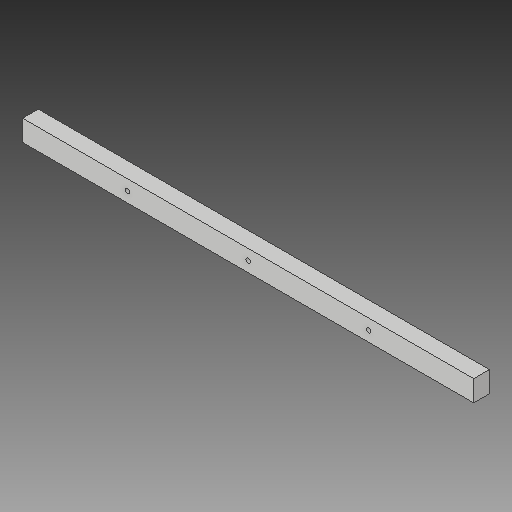
# Autodesk Inventor part: Wiper Springloaded 1
Saved by Autodesk Inventor 2019 (Build 230136000, 136)
## iProperties
Created: 2020-03-14
Part Number: Wiper Springloaded 1
Material: Generic
Document SubType Name: Modeling
Designer: Vijay
Density: 1 g/cm^3
Appearance: Default
Author: Vijay
Autodesk Inventor part; units mm, degrees
ref_plane "YZ Plane" through (0, 0, 0) normal (1, 0, 0) x (0, 1, 0)
ref_plane "XZ Plane" through (0, 0, 0) normal (0, 1, 0) x (-1, 0, 0)
ref_plane "XY Plane" through (0, 0, 0) normal (0, 0, 1) x (1, 0, 0)
sketch "Sketch1" plane through (0, 0, 0) normal (0, 0, 1) x (1, 0, 0)
  line L0 (-212.4247, -46.9955) -> (-212.4247, -61.9955) projected
  line L1 (-212.4247, -61.9955) -> (213.9753, -61.9955) projected
  line L2 (213.9753, -61.9955) -> (213.9753, -46.9955) projected
  line L3 (213.9753, -46.9955) -> (-212.4247, -46.9955) projected
  line L4 (213.9754, 278.5874) -> (243.9754, 278.5874) projected
  line L5 (243.9754, 278.5874) -> (243.9753, -71.9955) projected
  line L6 (243.9753, -71.9955) -> (-242.4247, -71.9955) projected
  line L7 (-242.4247, -71.9955) -> (-242.4246, 278.5875) projected
  line L8 (-242.4246, 278.5875) -> (-212.4246, 278.5875) projected
  line L9 (-212.4246, 278.5875) -> (-212.4247, -21.9955) projected
  line L10 (-212.4247, -21.9955) -> (213.9753, -21.9955) projected
  line L11 (213.9753, -21.9955) -> (213.9754, 278.5874) projected
  line L12 (-217.4247, -3.4496) -> (212.5753, -3.4496)
  line L13 (212.5753, -3.4496) -> (212.5753, 16.5504)
  line L14 (212.5753, 16.5504) -> (-217.4247, 16.5504)
  line L15 (-217.4247, 16.5504) -> (-217.4247, -3.4496)
  point P0 (0, 0)
  dimension "d1" = 20
  dimension "d11" = 430
  constraints: 8 end point, 2 parallel, 1 horizontal, 1 perpendicular
  measures "d1" distance between parallel lines of L14 L12
  measures "d11" distance of L13.end L14.end
extrude "Extrusion1" add sketch "Sketch1" along normal blind 15 contours L12 L15 L14 L9 | L9 L14 L13 L12
sketch "Sketch2" plane through (0, 0, 0) normal (0, 0, -1) x (-1, 0, 0)
  line L0 (217.4247, -3.4496) -> (-212.5753, -3.4496) construction
  line L1 (2.4247, -3.4496) -> (2.4247, 18.0985) construction
  line L2 (217.4247, 16.5504) -> (217.4247, -3.4496) construction
  line L3 (217.4247, 6.5504) -> (-212.5753, 6.5504) construction
  line L4 (-212.5753, -3.4496) -> (-212.5753, 16.5504) construction
  circle A0 centre (117.4247, 6.5504) radius 2.1
  circle A1 centre (-112.5753, 6.5504) radius 2.1
  circle A2 centre (2.4247, 6.5504) radius 2.1
  point P0 (0, 0)
  dimension "d4" = 4.2
  dimension "d5" = 100
  dimension "d6" = 4.2
  dimension "d7" = 100
  dimension "d8" = 4.2
  constraints: 4 end point, 4 midpoint, 3 centre point, 2 point on line, 1 vertical
  measures "d4" diameter of A0
  measures "d5" distance from line of L2 A0.centre
  measures "d6" diameter of A1
  measures "d7" distance from line of A1.centre L4
  measures "d8" diameter of A2
extrude "Extrusion2" cut sketch "Sketch2" against normal through all
body "Solid1"
